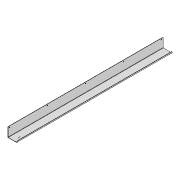
# Autodesk Inventor part: Dragchian_Holder
Saved by Autodesk Inventor 2020 (Build 240168000, 168)
## iProperties
Created: 2021-07-13
Part Number: Dragchian_Holder
Material: 一般
Document SubType Name: Sheet Metal
Designer: magnarecta
Density: 1 g/cm^3
Sheet Metal Rule: Default_mm
Appearance: 既定
Author: magnarecta
Autodesk Inventor part; units mm, degrees
ref_plane "YZ Plane" through (0, 0, 0) normal (1, 0, 0) x (0, 1, 0)
ref_plane "XZ Plane" through (0, 0, 0) normal (0, 1, 0) x (-1, 0, 0)
ref_plane "XY Plane" through (0, 0, 0) normal (0, 0, 1) x (1, 0, 0)
sketch "スケッチ1" plane through (0, 0, 0) normal (1, 0, 0) x (0, 1, 0)
  line L0 (0, 0) -> (60, 0)
  line L1 (60, 0) -> (60, 1000)
  line L2 (60, 1000) -> (0, 1000)
  line L3 (0, 1000) -> (0, 0)
  dimension "d0" = 60
  dimension "d1" = 1000
  measures "d0" distance of L0.start L0.end
  measures "d1" distance of L2.end L0.start
extrude "プレート1" add sketch "スケッチ1" along normal blind 1.5
sketch "スケッチ2" plane through (0, 1.5, 0) normal (0, -1, 0) x (1, 0, 0)
  line L0 (0, 1000) -> (0, 0)
  line L1 (0, 0) -> (60, 0)
  line L2 (60, 0) -> (60, 1000)
  line L3 (60, 1000) -> (0, 1000)
  constraints: 6 end point, 1 horizontal, 1 perpendicular, 1 vertical
edge flange "フランジ1" height 60 angle 90 thickness 1.5 bend radius 1.5 thickness toward (0, -1, 0) relief tear relief width 1.5 relief depth 0.75 edges at (1.5, 0, 500) wall of the first edge with corners at (0, 1.5, 1000) (0, 1.5, 0) (60, 1.5, 0) (60, 1.5, 1000)
bend "曲げ1"
corner "コーナー1"
sketch "スケッチ3" plane through (58.5, 0, 0) normal (1, 0, 0) x (0, 1, 0)
  line L0 (0, 1000) -> (0, 0)
  line L1 (0, 0) -> (10, 0)
  line L2 (10, 0) -> (10, 1000)
  line L3 (10, 1000) -> (0, 1000)
  constraints: 6 end point, 1 horizontal, 1 perpendicular, 1 vertical
edge flange "フランジ2" height 10 angle 90 thickness 1.5 bend radius 1.5 thickness toward (1, 0, 0) relief tear relief width 1.5 relief depth 0.75 edges at (60, 1.5, 500) wall of the first edge with corners at (58.5, 0, 1000) (58.5, 0, 0) (58.5, 10, 0) (58.5, 10, 1000)
bend "曲げ2"
corner "コーナー2"
fillet "フィレット1" radius 2 4 edges at (0.75, 60, 1000) (59.25, 10, 1000) (0.75, 60, 0) (59.25, 10, 0)
sketch "スケッチ4" plane through (1.5, 0, 0) normal (1, 0, 0) x (0, 0, -1)
  point P0 (0, 0)
sketch "スケッチ5" plane through (1.5, 0, 0) normal (1, 0, 0) x (0, 0, -1)
  line L0 (-998, 60) -> (-2, 60) projected
  line L1 (-1000, 3) -> (-1000, 58) projected
  line L2 (0, 58) -> (0, 3) projected
  point P0 (0, 0)
  point P1 (-990, 52)
  point P2 (-10, 52)
  point P3 (-745, 52)
  point P4 (-500, 52)
  point P5 (-255, 52)
  point P6 (-10, 52)
  dimension "d24" = 8
  dimension "d25" = 10
  dimension "d26" = 8
  dimension "d27" = 10
  dimension "d28" = 980
  dimension "d31" = 245
  constraints: 1 horizontal, 4 other
  measures "d24" distance from line of L0 point (-990, 52)
  measures "d25" distance from line of point (-990, 52) L1
  measures "d26" distance from line of point (-10, 52) L0
  measures "d27" distance from line of L2 point (-10, 52)
  measures "d28" distance of point (-990, 52) point (-10, 52)
  measures "d31" distance of point (-990, 52) point (-745, 52)
hole "穴1" at (1.5, 52, 990) at (1.5, 52, 10) at (1.5, 52, 745) at (1.5, 52, 500) at (1.5, 52, 255) direction (-1, 0, 0) diameter 5.2 depth 1.5 tip angle 118
sketch "スケッチ6" plane through (3, 1.5, 1000) normal (0, 1, 0) x (1, 0, 0)
  line L0 (57, 2) -> (57, 998) projected
  line L1 (0, 0) -> (54, 0) projected
  point P0 (-3, 1000)
  point P1 (34, 30)
  point P2 (34, 40)
  dimension "d43" = 10
  dimension "d44" = 23
  dimension "d45" = 30
  constraints: 1 vertical alignment
  measures "d43" distance of point (34, 40) point (34, 30)
  measures "d44" distance from line of point (34, 30) L0
  measures "d45" distance from line of point (34, 30) L1
hole "穴2" at (37, 1.5, 970) at (37, 1.5, 960) direction (0, -1, 0) diameter 3.242 depth 11.8 tip angle 118 thread size "M4x0.7" class "6H" standard "ISO Metric profile"
equation "\"d31\" = 0.25 * d28"
equation "\"d41\" = Thickness"
equation "\"d2\" = Thickness"
equation "\"d3\" = BendReliefWidth"
equation "\"d4\" = BendReliefDepth"
equation "\"d5\" = MinimumRemnant"
equation "\"d6\" = TransitionRadius"
equation "\"d9\" = BendRadius"
equation "\"d10\" = CornerReliefSize"
equation "\"d11\" = GapSize"
equation "\"d12\" = JacobiRadiusSize"
equation "\"d13\" = BendReliefWidth"
equation "\"d14\" = BendReliefDepth"
equation "\"d15\" = MinimumRemnant"
equation "\"d16\" = TransitionRadius"
equation "\"d19\" = BendRadius"
equation "\"d20\" = CornerReliefSize"
equation "\"d21\" = GapSize"
equation "\"d22\" = JacobiRadiusSize"
equation "\"BendRadius\" = Thickness"
equation "\"BendReliefWidth\" = Thickness"
equation "\"BendReliefDepth\" = 0.5 * Thickness"
equation "\"CornerReliefSize\" = 4 * Thickness"
equation "\"MinimumRemnant\" = 2 * Thickness"
equation "\"TransitionRadius\" = BendRadius"
equation "\"JacobiRadiusSize\" = BendRadius"
equation "\"GapSize\" = Thickness"
equation "\"Thickness\" = 1.5"
